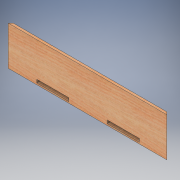
# Autodesk Inventor part: SkinnySideWidth
Saved by Autodesk Inventor 2016 (Build 200138000, 138)
## iProperties
Created: 2016-02-11
Part Number: SkinnySideWidth
Material: Wood (Birch)
Document SubType Name: Modeling
Designer: ron
Density: 0.55 g/cm^3
Appearance: Birch - Natural Polished
Mass: 828.134 g
Surface Area: 2264.58 cm^2
Volume: 1505.7 cm^3
Author: ron
Autodesk Inventor part; units mm, degrees
ref_plane "YZ Plane" through (0, 0, 0) normal (1, 0, 0) x (0, 1, 0)
ref_plane "XZ Plane" through (0, 0, 0) normal (0, 1, 0) x (-1, 0, 0)
ref_plane "XY Plane" through (0, 0, 0) normal (0, 0, 1) x (1, 0, 0)
sketch "Sketch1" plane through (0, 0, 0) normal (1, 0, 0) x (0, 1, 0)
  line L0 (0, 0) -> (155.1, 0)
  line L1 (155.1, 0) -> (155.1, -10)
  line L2 (0, -20) -> (0, 0)
  line L3 (155.1, -10) -> (101.6, -10)
  line L4 (101.6, -10) -> (101.6, -20)
  line L5 (101.6, -20) -> (0, -20)
  dimension "d0" = 53.5
  dimension "d1" = 155.1
  dimension "d2" = 10
  dimension "d3" = 10
  dimension "d4" = 20
  constraints: 12 end point, 3 horizontal, 2 parallel, 1 perpendicular
  measures "d0" distance of L1.end L3.end
  measures "d1" distance between parallel lines of L1 L2
  measures "d2" distance between parallel lines of L3 L5
  measures "d3" distance between parallel lines of L0 L3
  measures "d4" vertical distance of L4.end L0.end
extrude "Extrusion1" add sketch "Sketch1" along normal blind 629.2342
chamfer "Chamfer1" distance 19.812 angle 45 1 edges at (629.2342, 50.8, -20)
chamfer "Chamfer2" distance 19.812 angle 45 1 edges at (0, 50.8, -20)
sketch "Sketch2" plane through (609.4222, 0, -20) normal (0, 0, -1) x (-1, 0, 0)
  line L0 (589.6102, 0) -> (0, 0) projected
  line L1 (0, 0) -> (0, 6.35)
  line L2 (0, 0) -> (0, 101.6) projected
  line L3 (0, 6.35) -> (88.9, 6.35)
  line L4 (88.9, 6.35) -> (88.9, 26.35)
  line L5 (88.9, 26.35) -> (215.9, 26.35)
  line L6 (215.9, 26.35) -> (215.9, 6.35)
  line L7 (215.9, 6.35) -> (368.3, 6.35)
  line L8 (368.3, 6.35) -> (368.3, 19.05)
  line L9 (368.3, 19.05) -> (495.3, 19.05)
  line L10 (495.3, 19.05) -> (495.3, 6.35)
  line L11 (495.3, 6.35) -> (589.6102, 6.35)
  line L12 (589.6102, 101.6) -> (589.6102, 0) projected
  line L13 (88.9, 6.35) -> (215.9, 6.35)
  line L14 (368.3, 6.35) -> (495.3, 6.35)
  point P0 (609.4222, 0)
  dimension "d13" = 6.35
  dimension "d15" = 88.9
  dimension "d16" = 127
  dimension "d17" = 152.4
  dimension "d18" = 127
  dimension "d20" = 20
  dimension "d21" = 20
  dimension "d22" = 12.7
  dimension "d23" = 12.7
  constraints: 24 end point, 7 perpendicular, 2 horizontal, 2 point on line
  measures "d13" distance of L0.end L1.end
  measures "d15" distance of L1.end L3.end
  measures "d16" distance of L4.end L5.end
  measures "d17" distance of L6.end L7.end
  measures "d18" distance of L8.end L9.end
  measures "d20" distance of L3.end L4.end
  measures "d21" distance of L5.end L6.end
  measures "d22" distance of L7.end L8.end
  measures "d23" distance of L9.end L10.end
sketch "Sketch3" plane through (609.4222, 0, -20) normal (0, 0, -1) x (-1, 0, 0)
  line L0 (589.6102, 0) -> (0, 0)
  line L1 (0, 0) -> (0, 6.35)
  line L2 (0, 0) -> (0, 101.6)
  line L3 (0, 6.35) -> (88.9, 6.35)
  line L4 (88.9, 6.35) -> (88.9, 19.05)
  line L5 (88.9, 19.05) -> (215.9, 19.05)
  line L6 (215.9, 19.05) -> (215.9, 6.35)
  line L7 (215.9, 6.35) -> (368.3, 6.35)
  line L8 (368.3, 6.35) -> (368.3, 26.35)
  line L9 (368.3, 26.35) -> (495.3, 26.35)
  line L10 (495.3, 26.35) -> (495.3, 6.35)
  line L11 (495.3, 6.35) -> (589.6102, 6.35)
  line L12 (589.6102, 101.6) -> (589.6102, 0)
  line L13 (88.9, 6.35) -> (215.9, 6.35)
  line L14 (368.3, 6.35) -> (495.3, 6.35)
  line L15 (-19.812, 0) -> (0, 0) projected
  line L16 (0, 6.35) -> (0, 0)
  point P0 (609.4222, 0)
  point P1 (609.4222, 0)
  dimension "d24" = 6.35
  dimension "d25" = 88.9
  dimension "d26" = 127
  dimension "d27" = 152.4
  dimension "d28" = 127
  dimension "d29" = 12.7
  dimension "d30" = 12.7
  dimension "d31" = 20
  dimension "d32" = 20
  dimension "d37" = 6.35
  constraints: 32 end point, 7 perpendicular, 2 horizontal, 2 point on line, 1 vertical
  measures "d24" distance of L0.end L1.end
  measures "d25" distance of L1.end L3.end
  measures "d26" distance of L4.end L5.end
  measures "d27" distance of L6.end L7.end
  measures "d28" distance of L8.end L9.end
  measures "d29" distance of L3.end L4.end
  measures "d30" distance of L5.end L6.end
  measures "d31" distance of L7.end L8.end
  measures "d32" distance of L9.end L10.end
  measures "d37" distance of L1.end L15.end
extrude "Extrusion2" cut sketch "Sketch3" against normal blind 508 contours L4 L5 L6 L13
extrude "Extrusion3" cut sketch "Sketch2" against normal blind 508 contours L14 L8 L9 L10
body "Solid1"
